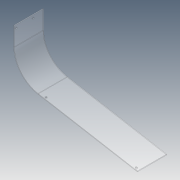
# Autodesk Inventor part: GE-12086-02
Saved by Autodesk Inventor 2012 (Build 160160000, 160)
## iProperties
Created: 2011-10-10
Part Number: GE-12086-02
Document SubType Name: Modeling
Designer: dfoster
Density: 1 g/cm^3
Description: Bottom
Material: Default
Title: Bottom
Author: dfoster
Autodesk Inventor part; units mm, degrees
ref_plane "YZ Plane" through (0, 0, 0) normal (1, 0, 0) x (0, 1, 0)
ref_plane "XZ Plane" through (0, 0, 0) normal (0, 1, 0) x (-1, 0, 0)
ref_plane "XY Plane" through (0, 0, 0) normal (0, 0, 1) x (1, 0, 0)
sketch "Sketch1" plane through (0, 0, 0) normal (0, 0, 1) x (1, 0, 0)
  line L0 (-89.1004, -3.8352) -> (336.0988, -78.8093) projected
  line L1 (336.0988, -75.5853) -> (336.0988, -78.8093) projected
  line L2 (336.0988, -75.5853) -> (-88.549, -0.7084) projected
  line L3 (-183.001, 111.8551) -> (-183.001, 183.0419) projected
  line L4 (-186.176, 183.0419) -> (-183.001, 183.0419) projected
  line L5 (-186.176, 183.0419) -> (-186.176, 111.8551) projected
  arc A0 (-186.176, 111.8551) -> (-89.1004, -3.8352) centre (-68.701, 111.8551) ccw projected
  arc A1 (-183.001, 111.8551) -> (-88.549, -0.7084) centre (-68.701, 111.8551) ccw projected
  point P0 (0, 0)
extrude "Extrusion1" add sketch "Sketch1" along normal blind 117.475
hole "Hole1" at (-186.176, 170.3419, 109.5375) direction (1, 0, 0) diameter 6.731 depth 25.4 tip angle 118
pattern_linear "Rectangular Pattern1" count 2 spacing 68.2625 along (0, 0, -1) of "Hole1"
hole "Hole2" at (323.5917, -76.6039, 109.5375) direction (0.1736482, 0.9848078, 0) diameter 6.731 depth 25.4 tip angle 118
pattern_linear "Rectangular Pattern2" count 2 spacing 368.3 along (-0.9848078, 0.1736482, 0) of "Hole2"
body "Solid1"
